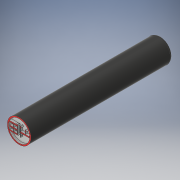
# Autodesk Inventor part: ueda_hanko
Saved by Autodesk Inventor 2019 (Build 230136000, 136)
## iProperties
Created: 2020-10-19
Part Number: ueda_hanko
Material: 一般
Document SubType Name: Modeling
Designer: Masato
Density: 1 g/cm^3
Appearance: 既定
Author: Masato
## iProperties of the stored document ueda_hanko_3D プリント.ipt
Created: 2020-10-19
Part Number: ueda_hanko_3D プリント
Material: 一般
Document SubType Name: Modeling
Designer: Masato
Density: 1 g/cm^3
Appearance: 既定
Author: Masato
Autodesk Inventor part; units mm, degrees
ref_plane "YZ Plane" through (0, 0, 0) normal (1, 0, 0) x (0, 1, 0)
ref_plane "XZ Plane" through (0, 0, 0) normal (0, 1, 0) x (-1, 0, 0)
ref_plane "XY Plane" through (0, 0, 0) normal (0, 0, 1) x (1, 0, 0)
sketch "スケッチ1" plane through (0, 0, 0) normal (0, 0, 1) x (1, 0, 0)
  circle A0 centre (0, 0) radius 5
  circle A1 centre (0, 0) radius 4.5
  dimension "d0" = 10
  dimension "d10" = 9
  constraints: 2 centre point, 2 coincident
  measures "d0" diameter of A0
  measures "d10" diameter of A1
ref_plane "作業平面1" through (0, 0, 0) normal (0, 0, -1) x (-1, 0, 0)
sketch "スケッチ2" plane through (0, 0, 0) normal (0, 0, -1) x (-1, 0, 0)
  line L0 (-5.5874, 2.4478) -> (5.5874, 2.4478) construction
  line L1 (5.5874, 2.4478) -> (5.5874, -2.4478) construction
  line L2 (5.5874, -2.4478) -> (-5.5874, -2.4478) construction
  line L3 (-5.5874, -2.4478) -> (-5.5874, 2.4478) construction
  line L4 (5.5874, 2.4478) -> (-5.5874, -2.4478) construction
  line L5 (5.5874, -2.4478) -> (-5.5874, 2.4478) construction
  line L6 (-2.6039, 0.0543) -> (-0.5793, 0.0543)
  line L7 (-0.5793, 0.0543) -> (-0.5793, 1.222)
  spline S0 degree 2 poles (-0.5793, 1.222) (-0.9655, 1.5328) (-0.9655, 1.5901) knots 0 0 0 1 1 1
  spline S1 degree 2 poles (-0.9655, 1.5901) (-0.9655, 1.6414) (-0.697, 1.9703) knots 0 0 0 1 1 1
  spline S2 degree 2 poles (-0.697, 1.9703) (-0.5612, 2.1392) (-0.5159, 2.1392) knots 0 0 0 1 1 1
  spline S3 degree 2 poles (-0.5159, 2.1392) (-0.4677, 2.1392) (-0.4677, 2.0759) knots 0 0 0 1 1 1
  line L8 (-0.4677, 2.0759) -> (-0.4677, -1.6263)
  spline S4 degree 2 poles (-0.4677, -1.6263) (-0.4677, -1.8888) (-0.4405, -2.0849) knots 0 0 0 1 1 1
  line L9 (-0.4405, -2.0849) -> (-0.6155, -2.1392)
  spline S5 degree 2 poles (-0.6155, -2.1392) (-0.5793, -1.8677) (-0.5793, -1.6293) knots 0 0 0 1 1 1
  line L10 (-0.5793, -1.6293) -> (-0.5793, -0.4375)
  line L11 (-0.5793, -0.4375) -> (-3.7746, -0.4375)
  spline S6 degree 2 poles (-3.7746, -0.4375) (-4.2151, -0.4375) (-4.4504, -0.4677) knots 0 0 0 1 1 1
  spline S7 degree 2 poles (-4.4504, -0.4677) (-4.4142, -0.0151) (-4.3659, 0.1328) knots 0 0 0 1 1 1
  spline S8 degree 2 poles (-4.3659, 0.1328) (-4.3388, 0.2233) (-4.2935, 0.2233) knots 0 0 0 1 1 1
  spline S9 degree 2 poles (-4.2935, 0.2233) (-4.2151, 0.2233) (-4.1578, 0.0543) knots 0 0 0 1 1 1
  line L12 (-4.1578, 0.0543) -> (-2.7155, 0.0543)
  line L13 (-2.7155, 0.0543) -> (-2.7155, 0.8388)
  spline S10 degree 2 poles (-2.7155, 0.8388) (-3.0927, 1.1284) (-3.0927, 1.1888) knots 0 0 0 1 1 1
  spline S11 degree 2 poles (-3.0927, 1.1888) (-3.0927, 1.2401) (-2.8302, 1.5539) knots 0 0 0 1 1 1
  spline S12 degree 2 poles (-2.8302, 1.5539) (-2.6944, 1.7138) (-2.6522, 1.7138) knots 0 0 0 1 1 1
  spline S13 degree 2 poles (-2.6522, 1.7138) (-2.6039, 1.7138) (-2.6039, 1.6504) knots 0 0 0 1 1 1
  line L14 (-2.6039, 1.6504) -> (-2.6039, 0.0543)
  line L15 (4.1034, -1.4) -> (4.2905, -1.4)
  spline S14 degree 2 poles (4.2905, -1.4) (4.4836, -1.4) (4.4836, -1.6866) knots 0 0 0 1 1 1
  spline S15 degree 2 poles (4.4836, -1.6866) (4.4836, -1.8797) (4.3237, -1.8797) knots 0 0 0 1 1 1
  spline S16 degree 2 poles (4.3237, -1.8797) (3.4487, -1.8526) (1.9763, -1.8526) knots 0 0 0 1 1 1
  spline S17 degree 2 poles (1.9763, -1.8526) (1.0651, -1.8526) (0.4164, -1.8767) knots 0 0 0 1 1 1
  spline S18 degree 2 poles (0.4164, -1.8767) (0.5341, -1.5961) (0.6879, -1.3276) knots 0 0 0 1 1 1
  line L16 (0.6879, -1.3276) -> (0.6879, 1.3185)
  spline S19 degree 2 poles (0.6879, 1.3185) (0.4466, 1.5358) (0.4466, 1.5901) knots 0 0 0 1 1 1
  spline S20 degree 2 poles (0.4466, 1.5901) (0.4466, 1.6414) (0.6397, 1.8677) knots 0 0 0 1 1 1
  spline S21 degree 2 poles (0.6397, 1.8677) (0.7392, 1.9823) (0.7875, 1.9823) knots 0 0 0 1 1 1
  spline S22 degree 2 poles (0.7875, 1.9823) (0.8478, 1.9823) (0.9444, 1.8405) knots 0 0 0 1 1 1
  line L17 (0.9444, 1.8405) -> (1.4935, 1.8405)
  spline S23 degree 2 poles (1.4935, 1.8405) (2.9237, 1.8405) (4.2573, 1.8737) knots 0 0 0 1 1 1
  spline S24 degree 2 poles (4.2573, 1.8737) (4.4685, 1.8737) (4.4685, 1.575) knots 0 0 0 1 1 1
  spline S25 degree 2 poles (4.4685, 1.575) (4.4685, 1.3728) (4.3056, 1.3728) knots 0 0 0 1 1 1
  line L18 (4.3056, 1.3728) -> (4.1034, 1.3728)
  line L19 (4.1034, 1.3728) -> (4.1034, -1.4)
  line L20 (3.9948, 1.3728) -> (2.3776, 1.3728)
  line L21 (2.3776, 1.3728) -> (2.3776, 0.1901)
  line L22 (2.3776, 0.1901) -> (3.9948, 0.1901)
  line L23 (3.9948, 0.1901) -> (3.9948, 1.3728)
  line L24 (2.3776, -1.4) -> (3.9948, -1.4)
  line L25 (3.9948, -1.4) -> (3.9948, -0.2685)
  line L26 (3.9948, -0.2685) -> (2.3776, -0.2685)
  line L27 (2.3776, -0.2685) -> (2.3776, -1.4)
  line L28 (2.269, 1.3728) -> (0.7996, 1.3728)
  line L29 (0.7996, 1.3728) -> (0.7996, 0.1901)
  line L30 (0.7996, 0.1901) -> (2.269, 0.1901)
  line L31 (2.269, 0.1901) -> (2.269, 1.3728)
  line L32 (2.269, -1.4) -> (2.269, -0.2685)
  line L33 (2.269, -0.2685) -> (0.7996, -0.2685)
  line L34 (0.7996, -0.2685) -> (0.7996, -1.4)
  line L35 (0.7996, -1.4) -> (2.269, -1.4)
  point P0 (0, 0)
  point P1 (0, 0)
  constraints: 4 end point, 1 coincident, 1 midpoint, 3 other
extrude "押し出し5" add sketch "スケッチ1" against normal blind 1
sketch "スケッチ3" plane through (0, 0, -1) normal (0, 0, -1) x (-1, 0, 0)
  circle A0 centre (0, 0) radius 5
  constraints: 1 centre point, 1 coincident
extrude "押し出し6" add sketch "スケッチ3" along normal blind 59
fillet "フィレット2" radius 1 1 edges at (5, 0, -60)
extrude "押し出し8" add sketch "スケッチ2" along normal blind 1
